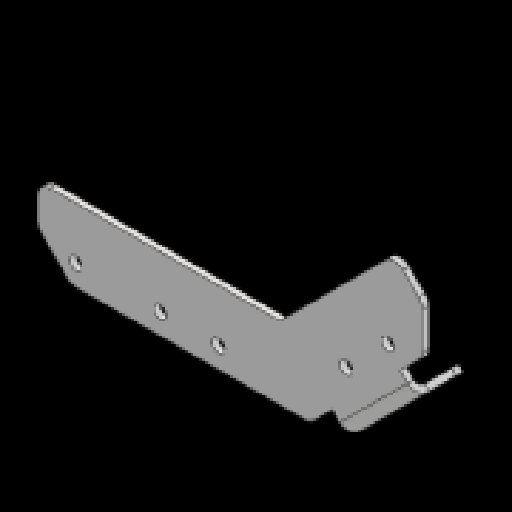
# Autodesk Inventor part: Part1
Saved by Autodesk Inventor 2025.2 (Build 292293000, 293)
## iProperties
Created: 2026-06-08
Part Number: Part1
Material: Generic
Document SubType Name: Sheet Metal
Designer: valer
Density: 1 g/cm^3
Sheet Metal Rule: Default
Appearance: Default
Author: valer
Autodesk Inventor part; units mm, degrees
ref_plane "YZ Plane" through (0, 0, 0) normal (1, 0, 0) x (0, 1, 0)
ref_plane "XZ Plane" through (0, 0, 0) normal (0, 1, 0) x (-1, 0, 0)
ref_plane "XY Plane" through (0, 0, 0) normal (0, 0, 1) x (1, 0, 0)
sketch "Sketch1" plane through (0, 0, 0) normal (0, 0, 1) x (1, 0, 0)
  arc A0 (-57.2353, -17.8992) -> (-52.9926, -16.1418) centre (-57.2353, -11.8992) ccw
  line L0 (-40.5074, -3.6566) -> (-52.9926, -16.1418)
  arc A1 (-40.5074, -3.6566) -> (-38.75, 0.5861) centre (-44.75, 0.5861) ccw
  line L1 (-38.75, 11.0048) -> (-38.75, 0.5861)
  line L2 (38.75, 17.1008) -> (-38.75, 17.1008)
  arc A2 (-38.75, 0.5861) -> (-36.9926, -3.6566) centre (-32.75, 0.5861) ccw
  line L3 (-24.5074, -16.1418) -> (-36.9926, -3.6566)
  arc A3 (-24.5074, -16.1418) -> (-20.2647, -17.8992) centre (-20.2647, -11.8992) ccw
  line L4 (20.2647, -17.8992) -> (-20.2647, -17.8992)
  arc A4 (20.2647, -17.8992) -> (24.5074, -16.1418) centre (20.2647, -11.8992) ccw
  line L5 (36.9926, -3.6566) -> (24.5074, -16.1418)
  arc A5 (36.9926, -3.6566) -> (38.75, 0.5861) centre (32.75, 0.5861) ccw
  line L6 (38.75, 11.0048) -> (38.75, 0.5861)
  line L7 (38.75, 11.0048) -> (-38.75, 11.0048)
  line L8 (-38.75, 0.5861) -> (-38.75, 11.0048)
  line L9 (93.5508, 71.9016) -> (38.75, 17.1008)
  arc A6 (50.4277, 5.4231) -> (54.6703, 3.6658) centre (54.6703, 9.6658) ccw
  line L10 (72.3272, 3.6658) -> (54.6703, 3.6658)
  arc A7 (72.3272, 3.6658) -> (76.5698, 5.4231) centre (72.3272, 9.6658) ccw
  line L11 (105.2284, 34.0818) -> (76.5698, 5.4231)
  arc A8 (105.2284, 34.0818) -> (106.9858, 38.3244) centre (100.9858, 38.3244) ccw construction
  line L12 (106.9858, 55.9813) -> (106.9858, 38.3244)
  arc A9 (106.9858, 55.9813) -> (105.2284, 60.2239) centre (100.9858, 55.9813) ccw
  line L13 (97.8613, 67.591) -> (105.2284, 60.2239)
  line L14 (97.8613, 67.591) -> (43.0605, 12.7903)
  line L15 (50.4277, 5.4231) -> (43.0605, 12.7903)
  line L16 (93.5508, 71.9016) -> (97.8613, 67.591)
  line L17 (-57.2353, -17.8992) -> (-20.2647, -17.8992)
  line L18 (20.2647, -17.8992) -> (53.2475, -17.8992)
  line L19 (53.2475, -17.8992) -> (76.5698, 5.4231)
  line L20 (105.2284, 34.0818) -> (106.9858, 35.8391)
  line L21 (106.9858, 35.8391) -> (106.9858, 38.3244)
  line L22 (72.3272, 3.6658) -> (74.8124, 3.6658)
  line L23 (74.8124, 3.6658) -> (76.5698, 5.4231)
  line L24 (-57.2353, -17.8992) -> (-59.0147, -17.8992)
  arc A10 (-63.2574, -16.1418) -> (-59.0147, -17.8992) centre (-59.0147, -11.8992) ccw
  line L25 (-63.2574, -16.1418) -> (-75.7426, -3.6566)
  arc A11 (-77.5, 0.5861) -> (-75.7426, -3.6566) centre (-71.5, 0.5861) ccw
  line L26 (-77.5, 0.5861) -> (-77.5, 11.0048)
  line L27 (-77.5, 11.0048) -> (-77.5, 17.1008)
  line L28 (-77.5, 17.1008) -> (-38.75, 17.1008)
  point P0 (0, 0)
extrude "Plate1" add sketch "Sketch1" along normal blind 3
fillet "Fillet3" radius 6 4 edges at (-77.5, 17.1008, 1.5) (106.9858, 35.8391, 1.5) (53.2475, -17.8992, 1.5) (93.5508, 71.9016, 1.5)
sketch "Sketch3" plane through (0, 0, 3) normal (0, 0, 1) x (1, 0, 0)
  line L0 (106.9858, 35.8391) -> (53.2475, -17.8992)
  line L1 (96.3792, 25.2325) -> (99.9147, 21.697)
  line L2 (99.9147, 21.697) -> (67.3896, -10.8281)
  line L3 (67.3896, -10.8281) -> (63.8541, -7.2926)
  point P0 (0, 0)
  dimension "d6" = 15
  dimension "d7" = 15
  dimension "d8" = 5
  measures "d6" distance from line of L0.start L1
  measures "d7" distance from line of L0.end L3
  measures "d8" distance between parallel lines of L0 L2
sheet face with bend "Face2" sketch "Sketch3" thickness 3 toward (0, 0, -1) bend radius 3 relief straight relief width 3 relief depth 1.5
bend "Bend1"
sketch "Sketch4" plane through (102.0361, 19.5757, -3) normal (0.7071068, -0.7071068, 0) x (0.7071068, 0.7071068, 0)
  line L0 (-45.9975, 0) -> (0, 0)
  line L1 (0, 0) -> (0, 19)
  line L2 (0, 19) -> (-45.9975, 19)
  line L3 (-45.9975, 19) -> (-45.9975, 0)
  constraints: 6 end point, 1 horizontal, 1 perpendicular, 1 vertical
edge flange "Flange1" height 25 angle 90 thickness 3 bend radius 3 thickness toward (0.7071068, -0.7071068, 0) relief straight relief width 3 relief depth 1.5 edges at (83.6522, 5.4344, 3) wall of the first edge with corners at (69.5109, -12.9495, -3) (102.0361, 19.5757, -3) (102.0361, 19.5757, -22) (69.5109, -12.9495, -22)
bend "Bend2"
corner "Corner1"
fillet "Fillet4" radius 6 2 edges at (103.0967, 18.515, -22) (70.5716, -14.0101, -22)
sketch "Sketch7" plane through (0, 0, 3) normal (0, 0, 1) x (1, 0, 0)
  circle A0 centre (9.2378, -7.8992) radius 3
  circle A1 centre (-18.7622, -7.8992) radius 3
  point P0 (0, 0)
  constraints: 2 centre point, 4 other
extrude "Cut4" cut sketch "Sketch7" against normal through all
sketch "Sketch8" plane through (0, 0, 3) normal (0, 0, 1) x (1, 0, 0)
  circle A0 centre (90.3602, 33.3556) radius 3
  circle A1 centre (70.5612, 13.5566) radius 3
  point P0 (0, 0)
  constraints: 2 centre point, 4 other
extrude "Cut5" cut sketch "Sketch8" against normal through all
sketch "Sketch9" plane through (0, 0, 3) normal (0, 0, 1) x (1, 0, 0)
  circle A0 centre (-59.0147, -7.8992) radius 3
  point P0 (0, 0)
  constraints: 1 centre point, 2 other
extrude "Cut6" cut sketch "Sketch9" against normal through all
sketch "Sketch10" plane through (104.1574, 17.4543, -3) normal (0.7071068, -0.7071068, 0) x (-0.7071068, -0.7071068, 0)
  arc A0 (45.9975, 13) -> (39.9975, 19) centre (39.9975, 13) ccw construction
  arc A1 (45.9975, 13) -> (39.9975, 19) centre (39.9975, 13) ccw construction
  line L0 (39.9975, 19) -> (6, 19) construction
  arc A2 (6, 19) -> (0, 13) centre (6, 13) ccw construction
  line L1 (0, 0) -> (0, 13) construction
  line L2 (0, 0) -> (45.9975, 0) construction
  line L3 (45.9975, 0) -> (45.9975, 13) construction
  line L4 (0, 0) -> (0, 13) construction
  line L5 (0, 11) -> (45.9975, 11) construction
  line L6 (45.9975, 0) -> (45.9975, 13) construction
  circle A3 centre (37.9975, 11) radius 3
  line L7 (0, 0) -> (45.9975, 0) projected
  line L8 (22.9987, 0) -> (22.9987, 19) construction
  circle A4 centre (8, 11) radius 3
  point P0 (85.9925, -3)
  dimension "d54" = 8
  dimension "d55" = 6
  dimension "d56" = 8
  constraints: 4 end point, 3 point on line, 2 centre point, 2 midpoint, 1 parallel, 1 symmetric about line, 1 other
  measures "d54" distance between parallel lines of L5 L0
  measures "d55" diameter of A3
  measures "d56" distance from line of L6 A3.centre
extrude "Cut7" cut sketch "Sketch10" against normal through all
equation "\"d48\" = Thickness"
equation "\"d50\" = Thickness"
equation "\"d52\" = Thickness"
equation "\"d57\" = Thickness"
equation "\"d0\" = Thickness"
equation "\"d9\" = BendRadius"
equation "\"d10\" = BendReliefWidth"
equation "\"d12\" = MinimumRemnant"
equation "\"d11\" = BendReliefDepth"
equation "\"d13\" = TransitionRadius"
equation "\"d14\" = BendReliefWidth"
equation "\"d15\" = BendReliefDepth"
equation "\"d16\" = MinimumRemnant"
equation "\"d17\" = TransitionRadius"
equation "\"d20\" = BendRadius"
equation "\"d21\" = CornerReliefSize"
equation "\"d22\" = GapSize"
equation "\"d23\" = JacobiRadiusSize"
equation "\"BendRadius\" = Thickness"
equation "\"BendReliefWidth\" = Thickness"
equation "\"BendReliefDepth\" = 0.5 * Thickness"
equation "\"CornerReliefSize\" = 4 * Thickness"
equation "\"MinimumRemnant\" = 2 * Thickness"
equation "\"TransitionRadius\" = BendRadius"
equation "\"JacobiRadiusSize\" = BendRadius"
equation "\"GapSize\" = Thickness"
equation "\"Thickness\" = 3"
body "Solid1"
